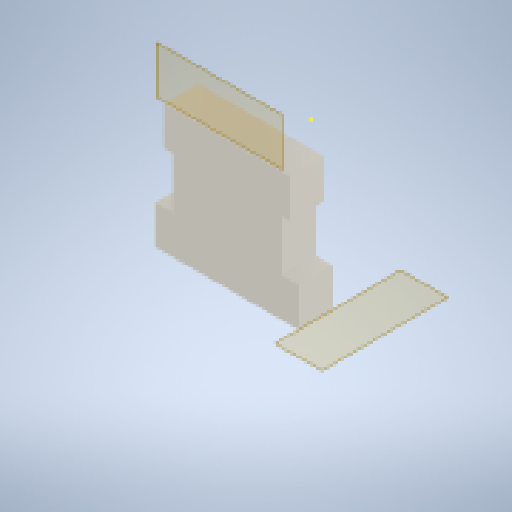
# Autodesk Inventor part: ОсноваКорпуса
Saved by Autodesk Inventor 2024.2 (Build 282272000, 272)
## iProperties
Created: 2025-03-03
Part Number: ОсноваКорпуса
Material: Титан
Document SubType Name: Modeling
Designer: Timofey
Density: 4.51 g/cm^3
Appearance: Титан
Mass: 21607.4 g
Surface Area: 10015 cm^2
Volume: 4791 cm^3
Author: Timofey
Autodesk Inventor part; units mm, degrees
ref_plane "YZ Plane" through (0, 0, 0) normal (1, 0, 0) x (0, 1, 0)
ref_plane "XZ Plane" through (0, 0, 0) normal (0, 1, 0) x (-1, 0, 0)
ref_plane "XY Plane" through (0, 0, 0) normal (0, 0, 1) x (1, 0, 0)
ref_plane "РабПлоскость1" through (519.783, -178.5074, 484.3845) normal (-0.0032, 1, 0.0035) x (-0.0024, 0.0035, -1)
sketch "Эскиз1" plane through (0, 0, 0) normal (0, 0, 1) x (-1, 0, 0)
  line L0 (0, 0) -> (0, 90)
  line L1 (0, 90) -> (-25, 90)
  line L2 (-25, 90) -> (-75, 90)
  line L3 (-75, 90) -> (-75, 540)
  line L4 (-75, 540) -> (425, 540)
  line L5 (425, 540) -> (425, 90)
  line L6 (425, 90) -> (-75, 90)
  line L7 (175, 315) -> (425, 315)
  line L8 (175, 315) -> (-75, 315)
  line L9 (425, 315) -> (425, 405)
  line L10 (425, 405) -> (365, 405)
  line L11 (365, 405) -> (365, 225)
  line L12 (365, 225) -> (425, 225)
  line L13 (-75, 315) -> (-75, 405)
  line L14 (-75, 405) -> (-15, 405)
  line L15 (-15, 405) -> (-15, 225)
  line L16 (-15, 225) -> (-75, 225)
  line L17 (0, 90) -> (0, 100)
  line L18 (0, 100) -> (-65, 100)
  line L19 (0, 100) -> (415, 100)
  line L20 (425, 540) -> (415, 540)
  line L21 (415, 530) -> (415, 100)
  line L22 (425, 540) -> (425, 530)
  line L23 (415, 530) -> (-65, 530)
  line L24 (-75, 540) -> (-65, 540)
  line L25 (-65, 530) -> (-65, 100)
  point P0 (415, 405)
  point P1 (-65, 405)
  point P2 (-65, 225)
  point P3 (415, 225)
  dimension "d0" = 90
  dimension "d1" = 25
  dimension "d2" = 50
  dimension "d3" = 450
  dimension "d4" = 500
  dimension "d5" = 90
  dimension "d6" = 60
  dimension "d7" = 180
  dimension "d8" = 60
  dimension "d35" = 10
  dimension "d36" = 10
  dimension "d37" = 10
  constraints: 52 end point, 14 perpendicular, 12 point on line, 2 midpoint, 2 vertical, 1 horizontal
  measures "d0" distance of L0.start L0.end
  measures "d1" distance of L0.end L1.end
  measures "d2" distance of L1.end L2.end
  measures "d3" distance of L2.end L3.end
  measures "d4" distance of L3.end L4.end
  measures "d5" distance of L7.end L9.end
  measures "d6" distance of L9.end L10.end
  measures "d7" distance of L10.end L11.end
  measures "d8" distance of L13.end L14.end
  measures "d35" distance of L4.end L20.end
  measures "d36" distance of L4.end L22.end
  measures "d37" distance of L3.end L24.end
ref_plane "РабПлоскость2" through (0, 0, 60) normal (0, 0, 1) x (1, 0, 0)
extrude "Выдавливание6" add sketch "Эскиз1" along normal mid plane 120 contours L17 L19 L21 L12 L5 L6 | L1 L2 L3 L16 L25 L18 L17 | L10 L21 L23 L25 L14 L3 L4 L5
sketch "Эскиз7" plane through (0, 0, 60) normal (0, 0, 1) x (1, 0, 0)
  line L0 (-415, -100) -> (65, -100) projected
  line L1 (-415, -100) -> (65, -100)
  line L2 (65, -225) -> (75, -225) projected
  line L3 (65, -100) -> (65, -225)
  line L4 (65, -225) -> (15, -225)
  line L5 (15, -225) -> (15, -405)
  line L6 (15, -405) -> (65, -405)
  line L7 (-415, -530) -> (65, -530) projected
  line L8 (65, -405) -> (65, -530)
  line L9 (65, -530) -> (-415, -530)
  line L10 (-415, -530) -> (-415, -405)
  line L11 (-415, -225) -> (-415, -100)
  line L12 (-415, -405) -> (-365, -405)
  line L13 (-365, -405) -> (-365, -225)
  line L14 (-365, -225) -> (-415, -225)
  point P0 (0, 0)
  dimension "d40" = 50
  dimension "d41" = 180
  dimension "d43" = 50
  constraints: 24 end point, 8 perpendicular, 2 horizontal, 2 point on line, 1 collinear
  measures "d40" distance of L2.start L4.end
  measures "d41" distance of L4.end L5.end
  measures "d43" distance of L10.end L12.end
extrude "Выдавливание7" add sketch "Эскиз7" against normal blind 10
sketch "Эскиз8" plane through (0, 0, 50) normal (0, 0, -1) x (-1, 0, 0)
  line L0 (415, -405) -> (415, -530) projected
  line L1 (365, -225) -> (365, -405) projected
  line L2 (415, -405) -> (365, -405)
  line L3 (365, -405) -> (365, -225)
  line L4 (415, -100) -> (415, -225) projected
  line L5 (365, -225) -> (415, -225)
  line L6 (415, -225) -> (415, -220)
  line L7 (415, -220) -> (355, -220)
  line L8 (355, -220) -> (355, -410)
  line L9 (355, -410) -> (415, -410)
  line L10 (415, -410) -> (415, -405)
  line L11 (425, -405) -> (425, -540) projected
  line L12 (-65, -225) -> (-65, -100) projected
  line L13 (-65, -225) -> (-15, -225) projected
  line L14 (-65, -225) -> (-15, -225)
  line L15 (-15, -225) -> (-15, -405)
  line L16 (-15, -405) -> (-65, -405)
  line L17 (-65, -405) -> (-65, -410)
  line L18 (-65, -410) -> (-5, -410)
  line L19 (-5, -410) -> (-5, -220)
  line L20 (-5, -220) -> (-65, -220)
  point P0 (0, 0)
  dimension "d46" = 5
  dimension "d47" = 60
  dimension "d48" = 190
  dimension "d49" = 5
  dimension "d50" = 60
  dimension "d51" = 190
  constraints: 30 end point, 9 perpendicular, 3 parallel, 3 point on line, 1 horizontal, 1 vertical
  measures "d46" distance of L4.end L6.end
  measures "d47" distance of L6.end L7.end
  measures "d48" distance of L7.end L8.end
  measures "d49" distance of L16.end L17.end
  measures "d50" distance of L17.end L18.end
  measures "d51" distance of L19.end L18.end
extrude "Выдавливание8" add sketch "Эскиз8" along normal blind 110
sketch "Эскиз9" plane through (0, 0, 50) normal (0, 0, -1) x (-1, 0, 0)
  line L0 (415, -100) -> (415, -220) projected
  line L1 (415, -100) -> (415, -95)
  line L2 (415, -95) -> (-65, -95)
  line L3 (-65, -220) -> (-65, -100) projected
  line L4 (-65, -95) -> (-65, -100)
  line L5 (-65, -100) -> (415, -100)
  point P0 (0, 0)
  dimension "d54" = 5
  constraints: 8 end point, 2 perpendicular, 1 parallel, 1 vertical
  measures "d54" distance of L0.start L1.end
extrude "Выдавливание9" cut sketch "Эскиз9" along normal blind 110
sketch "Эскиз10" plane through (0, 0, 50) normal (0, 0, -1) x (-1, 0, 0)
  line L0 (415, -410) -> (415, -427.5)
  line L1 (415, -410) -> (415, -530) projected
  line L2 (415, -427.5) -> (-65, -427.5)
  line L3 (-65, -530) -> (-65, -410) projected
  line L4 (-65, -427.5) -> (-65, -410)
  line L5 (-5, -410) -> (-5, -220) projected
  line L6 (-65, -410) -> (-5, -410)
  line L7 (-5, -410) -> (-5, -417.5)
  line L8 (-5, -417.5) -> (355, -417.5)
  line L9 (355, -410) -> (415, -410) projected
  line L10 (355, -417.5) -> (355, -410)
  line L11 (355, -410) -> (415, -410)
  point P0 (0, 0)
  dimension "d57" = 17.5
  dimension "d58" = 480
  dimension "d59" = 7.5
  constraints: 16 end point, 4 perpendicular, 1 collinear, 1 parallel, 1 point on line
  measures "d57" distance of L0.start L0.end
  measures "d58" distance of L0.end L2.end
  measures "d59" distance of L5.start L7.end
extrude "Выдавливание10" add sketch "Эскиз10" along normal blind 110
sketch "Эскиз11" plane through (0, 0, 50) normal (0, 0, -1) x (-1, 0, 0)
  line L0 (355, -220) -> (355, -417.5) projected
  line L1 (355, -220) -> (355, -260)
  line L2 (355, -260) -> (-5, -260)
  line L3 (-5, -220) -> (-5, -417.5) projected
  line L4 (-5, -260) -> (-5, -250)
  line L5 (-5, -250) -> (355, -250)
  point P0 (0, 0)
  dimension "d62" = 40
  dimension "d63" = 10
  constraints: 8 end point, 4 point on line, 2 perpendicular
  measures "d62" distance of L0.start L1.end
  measures "d63" distance of L2.end L4.end
extrude "Выдавливание11" add sketch "Эскиз11" along normal blind 110
sketch "Эскиз12" plane through (0, 0, 60) normal (0, 0, 1) x (1, 0, 0)
  line L0 (15, -225) -> (75, -225) projected
  line L1 (75, -90) -> (-425, -90) projected
  line L2 (75, -225) -> (45, -225)
  line L3 (45, -225) -> (45, -90)
  line L4 (45, -90) -> (75, -90)
  line L5 (75, -90) -> (75, -225)
  line L6 (-425, -225) -> (-365, -225) projected
  line L7 (-425, -225) -> (-395, -225)
  line L8 (-395, -225) -> (-395, -90)
  line L9 (-395, -90) -> (-425, -90)
  line L10 (-425, -90) -> (-425, -225)
  point P0 (0, 0)
  dimension "d66" = 30
  constraints: 16 end point, 4 parallel, 2 horizontal, 2 perpendicular, 2 point on line
  measures "d66" distance of L3.end L4.end
extrude "Выдавливание12" cut sketch "Эскиз12" against normal blind 120
sketch "Эскиз13" plane through (0, 0, 50) normal (0, 0, -1) x (-1, 0, 0)
  line L0 (-45, -95) -> (-45, -220) projected
  line L1 (395, -95) -> (-45, -95) projected
  line L2 (-45, -220) -> (-35, -220)
  line L3 (-35, -220) -> (-35, -95)
  line L4 (-35, -95) -> (-45, -95)
  line L5 (-45, -95) -> (-45, -220)
  line L6 (395, -95) -> (385, -95)
  line L7 (385, -95) -> (385, -220)
  line L8 (385, -220) -> (395, -220)
  line L9 (395, -220) -> (395, -95)
  point P0 (0, 0)
  dimension "d69" = 10
  dimension "d70" = 10
  constraints: 16 end point, 4 parallel, 2 horizontal, 2 perpendicular, 2 point on line
  measures "d69" distance of L4.end L3.end
  measures "d70" distance of L8.end L7.end
extrude "Выдавливание13" add sketch "Эскиз13" along normal blind 110
sketch "Эскиз14" plane through (0, 0, -60) normal (0, 0, -1) x (-1, 0, 0)
  point P0 (0, 0)
sketch "Эскиз15" plane through (75, -540, 60) normal (1, 0, 0) x (0, 0, -1)
  line L0 (0, 135) -> (0, 0) projected
  line L1 (120, 0) -> (120, 135) projected
  line L2 (0, 0) -> (120, 0)
  line L3 (120, 0) -> (60, 0)
  arc A0 (45, 0) -> (75, 0) centre (60, 0) ccw
  point P0 (60, 540)
  dimension "d73" = 60
  dimension "d74" = 30
  constraints: 4 end point, 2 point on circle, 2 point on line, 1 centre point, 1 coincident, 1 midpoint, 1 perpendicular
  measures "d73" distance of L1.start L3.end
  measures "d74" diameter of A0
extrude "Выдавливание14" add sketch "Эскиз15" against normal blind 500
sketch "Эскиз16" plane through (0, 0, 50) normal (0, 0, -1) x (-1, 0, 0)
  line L0 (-35, -220) -> (-35, -95) projected
  line L1 (-35, -220) -> (-35, -215)
  line L2 (-35, -215) -> (-5, -215)
  line L3 (-5, -220) -> (-35, -220) projected
  line L4 (-5, -215) -> (-5, -220)
  line L5 (-5, -220) -> (-35, -220)
  line L6 (385, -220) -> (355, -220) projected
  line L7 (355, -220) -> (355, -215)
  line L8 (355, -215) -> (385, -215)
  line L9 (385, -95) -> (385, -220) projected
  line L10 (385, -215) -> (385, -220)
  line L11 (355, -220) -> (385, -220)
  point P0 (0, 0)
  dimension "d77" = 5
  constraints: 16 end point, 5 perpendicular, 2 point on line, 1 collinear, 1 vertical
  measures "d77" distance of L0.start L1.end
extrude "Выдавливание15" add sketch "Эскиз16" along normal blind 110
